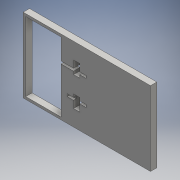
# Autodesk Inventor part: Lag2-3
Saved by Autodesk Inventor 2016 (Build 200138000, 138)
## iProperties
Created: 2016-12-12
Part Number: Lag2-3
Material: Generic
Document SubType Name: Modeling
Designer: Simon
Density: 1 g/cm^3
Appearance: Default
Author: Simon
Autodesk Inventor part; units mm, degrees
ref_plane "YZ Plane" through (0, 0, 0) normal (1, 0, 0) x (0, 1, 0)
ref_plane "XZ Plane" through (0, 0, 0) normal (0, 1, 0) x (-1, 0, 0)
ref_plane "XY Plane" through (0, 0, 0) normal (0, 0, 1) x (1, 0, 0)
sketch "Sketch1" plane through (0, 0, 0) normal (0, 1, 0) x (-1, 0, 0)
  line L0 (-50.5, -29.5) -> (50.5, -29.5)
  line L1 (50.5, -29.5) -> (50.5, 29.5)
  line L2 (50.5, 29.5) -> (-50.5, 29.5)
  line L3 (-50.5, 29.5) -> (-50.5, -29.5)
  line L4 (-50.5, -29.5) -> (50.5, 29.5) construction
  line L5 (50.5, -29.5) -> (-50.5, 29.5) construction
  line L6 (48.5, 27.5) -> (20.5, 27.5)
  line L7 (20.5, 27.5) -> (20.5, -27.5)
  line L8 (20.5, -27.5) -> (48.5, -27.5)
  line L9 (48.5, -27.5) -> (48.5, 27.5)
  line L10 (48.5, 27.5) -> (48.5, 29.5)
  line L11 (48.5, -27.5) -> (48.5, -29.5)
  line L12 (48.5, -27.5) -> (50.5, -27.5)
  line L13 (15.5, -9) -> (15.5, -11)
  line L14 (15.5, -11) -> (10.5, -11)
  line L15 (15.5, -9) -> (10.5, -9)
  line L16 (15.5, -10) -> (10.5, -10)
  line L17 (10.5, 16.6667) -> (10.5, 13.3333)
  line L18 (10.5, 13.3333) -> (10.5, 10)
  line L19 (10.5, 10) -> (10.5, 6.6667)
  line L20 (10.5, 6.6667) -> (5.5, 6.6667)
  line L21 (5.5, 6.6667) -> (5.5, 16.6667)
  line L22 (5.5, 16.6667) -> (10.5, 16.6667)
  line L23 (10.5, -6.6667) -> (5.5, -6.6667)
  line L24 (5.5, -6.6667) -> (5.5, -16.6667)
  line L25 (5.5, -16.6667) -> (10.5, -16.6667)
  line L26 (10.5, 6.6667) -> (10.5, -6.6667)
  line L27 (10.5, -6.6667) -> (10.5, -10)
  line L28 (10.5, -10) -> (10.5, -13.3333)
  line L29 (10.5, -13.3333) -> (10.5, -16.6667)
  line L30 (50.5, 0) -> (-50.5, 0)
  line L31 (20.5, 9) -> (20.5, 11)
  line L32 (20.5, 11) -> (10.5, 11)
  line L33 (20.5, 9) -> (10.5, 9)
  line L34 (20.5, 10) -> (10.5, 10)
  line L35 (0.5, 11) -> (0.5, 9)
  line L36 (0.5, 9) -> (5.5, 9)
  line L37 (0.5, 11) -> (5.5, 11)
  line L38 (0.5, -9) -> (0.5, -11)
  line L39 (0.5, -11) -> (5.5, -11)
  line L40 (0.5, -9) -> (5.5, -9)
  line L41 (20.5, 11) -> (10.5, 11)
  line L42 (10.5, 11) -> (10.5, 9)
  line L43 (10.5, 9) -> (20.5, 9)
  line L44 (20.5, 9) -> (20.5, 11)
  point P0 (0, 0)
  point P1 (10.5, 0)
  dimension "d0" = 101
  dimension "d1" = 59
  dimension "d2" = 2
  dimension "d3" = 28
  dimension "d4" = 10
  dimension "d5" = 5
  dimension "d6" = 20
  dimension "d7" = 2
  dimension "d8" = 10
  dimension "d9" = 5
  constraints: 90 end point, 20 equal length, 16 point on line, 15 perpendicular, 11 horizontal, 7 midpoint, 5 vertical, 3 collinear
  measures "d0" distance of L2.end L1.end
  measures "d1" distance of L1.end L0.end
  measures "d2" distance of L6.start L10.end
  measures "d3" distance of L7.end L8.end
  measures "d4" distance of L20.end L21.end
  measures "d5" distance of L21.end L17.start
  measures "d6" distance of L16.end L18.end
  measures "d7" distance of L31.start L31.end
  measures "d8" distance of L31.end L32.end
  measures "d9" distance of L13.end L14.end
extrude "Extrusion1" add sketch "Sketch1" along normal blind 2 contours L3 L30 L7 L8 L11 L0 | L11 L12 L1 L0 | L3 L2 L10 L6 L7 L32 L18 L17 L22 L21 L37 L35 L36 L20 L26 L30 | L9 L30 L1 L12 | L26 L19 L33 L7 L30 | L9 L10 L2 L1 L30
sketch "Sketch2" plane through (0, 2, 0) normal (0, 1, 0) x (1, 0, 0)
  line L0 (50.5, -29.5) -> (-50.5, -29.5)
  line L1 (-50.5, -29.5) -> (-50.5, 29.5)
  line L2 (-50.5, 29.5) -> (50.5, 29.5)
  line L3 (50.5, 29.5) -> (50.5, -29.5)
  line L4 (-10.5, -6.6667) -> (-5.5, -6.6667) projected
  line L5 (-5.5, -16.6667) -> (-10.5, -16.6667) projected
  line L6 (-5.5, -6.6667) -> (-10.5, -6.6667)
  line L7 (-10.5, -6.6667) -> (-10.5, -16.6667)
  line L8 (-10.5, -16.6667) -> (-5.5, -16.6667)
  line L9 (-5.5, -16.6667) -> (-5.5, -6.6667)
  line L10 (-20.5, -11) -> (-20.5, -27.5) projected
  line L11 (-20.5, -27.5) -> (-48.5, -27.5)
  line L12 (-48.5, -27.5) -> (-48.5, 27.5)
  line L13 (-48.5, 27.5) -> (-20.5, 27.5)
  line L14 (-20.5, 27.5) -> (-20.5, -27.5)
  line L15 (-5.5, 11) -> (-5.5, 16.6667) projected
  line L16 (-10.5, 9) -> (-10.5, 6.6667) projected
  line L17 (-5.5, 16.6667) -> (-10.5, 16.6667)
  line L18 (-10.5, 16.6667) -> (-10.5, 6.6667)
  line L19 (-10.5, 6.6667) -> (-5.5, 6.6667)
  line L20 (-5.5, 6.6667) -> (-5.5, 16.6667)
  line L21 (-10.5, -9) -> (-20.5, -9) projected
  line L22 (-20.5, -11) -> (-10.5, -11) projected
  line L23 (-10.5, -9) -> (-20.5, -9)
  line L24 (-20.5, -9) -> (-20.5, -11)
  line L25 (-20.5, -11) -> (-10.5, -11)
  line L26 (-10.5, -11) -> (-10.5, -9)
  point P0 (0, 0)
  constraints: 40 end point, 10 parallel, 5 horizontal, 5 perpendicular
extrude "Extrusion2" add sketch "Sketch2" along normal blind 3
body "Solid1"
